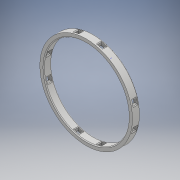
# Autodesk Inventor part: Attache centre
Saved by Autodesk Inventor 2017 (Build 210142000, 142)
## iProperties
Part Number: Attache centre
Material: Générique
Document SubType Name: Modeling
Designer: Thomas
Density: 1 g/cm^3
Appearance: Par défaut
Author: Thomas
Autodesk Inventor part; units mm, degrees
sketch "Esquisse1" plane through (0, 0, 0) normal (0, 1, 0) x (-1, 0, 0)
  line L0 (-42.5, 28) -> (42.5, 28) construction
  line L1 (42.5, 28) -> (42.5, -28) construction
  line L2 (42.5, -28) -> (-42.5, -28) construction
  line L3 (-42.5, -28) -> (-42.5, 28) construction
  line L4 (-42.5, 28) -> (42.5, -28) construction
  line L5 (42.5, 28) -> (-42.5, -28) construction
  circle A0 centre (0, 0) radius 60
  circle A1 centre (0, 0) radius 55
  line L6 (0, 0) -> (94, 94) construction
  line L7 (0, 0) -> (132.9361, 0) construction
  line L8 (0, 0) -> (-94, 94) construction
  line L9 (0, 0) -> (-94, -94) construction
  line L10 (0, 0) -> (94, -94) construction
  arc A2 (42.4264, 42.4264) -> (110, 0) centre (152.2245, 142.2782) ccw construction
  arc A3 (110, 0) -> (42.4264, -42.4264) centre (152.2245, -142.2782) ccw construction
  arc A4 (-42.4264, 42.4264) -> (0, 110) centre (-142.2782, 152.2245) ccw construction
  arc A5 (0, 110) -> (42.4264, 42.4264) centre (142.2782, 152.2245) ccw construction
  arc A6 (-42.4264, -42.4264) -> (-110, 0) centre (-152.2245, -142.2782) ccw construction
  arc A7 (-110, 0) -> (-42.4264, 42.4264) centre (-152.2245, 142.2782) ccw construction
  arc A8 (42.4264, -42.4264) -> (0, -110) centre (142.2782, -152.2245) ccw construction
  arc A9 (0, -110) -> (-42.4264, -42.4264) centre (-142.2782, -152.2245) ccw construction
  arc A10 (-57.9555, 15.5291) -> (-55, 95.2628) centre (-199.3288, 60.6911) ccw construction
  arc A11 (-55, 95.2628) -> (15.5291, 57.9555) centre (47.1043, 202.9694) ccw construction
  arc A12 (15.5291, -57.9555) -> (-55, -95.2628) centre (47.1043, -202.9694) ccw construction
  arc A13 (-55, -95.2628) -> (-57.9555, -15.5291) centre (-199.3288, -60.6911) ccw construction
  line L11 (0, 110) -> (0, 57.9555) construction
  line L12 (-55, -95.2628) -> (0, 0) construction
  line L13 (-55, 95.2628) -> (0, 0) construction
  line L14 (95.3744, -14.2176) -> (35.3744, 89.7054) construction
  line L15 (35.3744, 89.7054) -> (-95.3744, 14.2176) construction
  line L16 (-95.3744, 14.2176) -> (-35.3744, -89.7054) construction
  line L17 (-35.3744, -89.7054) -> (95.3744, -14.2176) construction
  line L18 (95.3744, -14.2176) -> (-95.3744, 14.2176) construction
  line L19 (35.3744, 89.7054) -> (-35.3744, -89.7054) construction
  dimension "d2" = 120
  dimension "d0" = 85
  dimension "d1" = 56
  dimension "d3" = 110
  dimension "d4" = 45
  dimension "d7" = 360
  dimension "d11" = 360
  dimension "d15" = 360
  constraints: 40 end point, 24 point on circle, 13 centre point, 4 midpoint, 4 parallel, 2 coincident, 2 horizontal, 2 perpendicular, 2 point on line, 2 symmetric about line, 1 equal length, 1 vertical, 68 other
  measures "d0" distance of L1.end L2.end
  measures "d1" distance of L0.end L1.end
  measures "d3" diameter of A1
  measures "d4" angle of L7 L6
extrude "Extrusion1" add sketch "Esquisse1" along normal blind 10
ref_plane "Plan de construction1" through (81, 0, 0) normal (1, 0, 0) x (0, 1, 0)
sketch "Esquisse2" plane through (81, 0, 0) normal (1, 0, 0) x (0, 1, 0)
  line L0 (8, 18.0155) -> (2, 18.0155)
  line L1 (2, 18.0155) -> (2, 12.0155)
  line L2 (2, 12.0155) -> (8, 12.0155)
  line L3 (8, 12.0155) -> (8, 18.0155)
  line L4 (8, 18.0155) -> (2, 12.0155) construction
  line L5 (2, 18.0155) -> (8, 12.0155) construction
  line L6 (10.0489, 0.0155) -> (-6.9511, 0.0155) construction
  line L7 (8, -17.9845) -> (2, -17.9845)
  line L8 (2, -17.9845) -> (2, -11.9845)
  line L9 (2, -11.9845) -> (8, -11.9845)
  line L10 (8, -11.9845) -> (8, -17.9845)
  point P0 (0, 0)
  point P1 (5, 15.0155)
  dimension "d22" = 15
  dimension "d26" = 6
  dimension "d27" = 6
  constraints: 22 end point, 4 symmetric about line, 2 horizontal, 2 midpoint, 2 parallel, 1 perpendicular
  measures "d22" distance from line of point (5, 15.015) L6
  measures "d26" distance of L1.end L2.end
  measures "d27" distance of L0.end L1.end
extrude "Extrusion2" cut sketch "Esquisse2" against normal blind 150
ref_plane "Plan de construction2" through (0, 0, 80) normal (0, 0, 1) x (1, 0, 0)
sketch "Esquisse3" plane through (0, 0, 80) normal (0, 0, 1) x (1, 0, 0)
  line L0 (-0.0028, -2.9025) -> (-0.0028, 13.0975) construction
  line L1 (-18.0028, 2) -> (-12.0028, 2)
  line L2 (-12.0028, 2) -> (-12.0028, 8)
  line L3 (-12.0028, 8) -> (-18.0028, 8)
  line L4 (-18.0028, 8) -> (-18.0028, 2)
  line L5 (17.9972, 2) -> (11.9972, 2)
  line L6 (11.9972, 2) -> (11.9972, 8)
  line L7 (11.9972, 8) -> (17.9972, 8)
  line L8 (17.9972, 8) -> (17.9972, 2)
  point P0 (0, 0)
  point P1 (-15.0028, 5)
  point P2 (14.9972, 5)
  dimension "d28" = 6
  dimension "d29" = 6
  dimension "d31" = 15
  dimension "d32" = 3
  dimension "d33" = 3
  constraints: 18 end point, 5 symmetric about line, 2 parallel, 1 horizontal, 1 perpendicular, 1 vertical
  measures "d28" distance of L2.end L3.end
  measures "d29" distance of L3.end L1.start
  measures "d31" distance from line of L0 point (-15.003, 5)
  measures "d32" distance from line of L2 point (-15.003, 5)
  measures "d33" distance from line of L3 point (-15.003, 5)
extrude "Extrusion3" cut sketch "Esquisse3" against normal blind 150
ref_plane "Plan de construction3" through (-35.3744, 0, 89.7054) normal (0.5, 0, 0.866) x (0, 1, 0)
sketch "Esquisse4" plane through (-35.3744, 0, 89.7054) normal (0.5, 0, 0.866) x (0, 1, 0)
  line L0 (0, -75.4878) -> (4, -75.4878) construction
  constraints: 2 end point, 1 horizontal
fillet "Congé1" radius 1 3 edges at (60, 10, 0) (55, 10, 0) (55, 0, 0)
fillet "Congé2" radius 1 32 edges at (-53.6715, 5, 12.0155) (53.6715, 5, 12.0155) (-58.7846, 5, 12.0155) (58.7846, 5, 12.0155) (-57.2315, 5, 18.0155) (57.2315, 5, 18.0155) (-51.9658, 5, 18.0155) (51.9658, 5, 18.0155) (53.6784, 5, -11.9845) (-53.6784, 5, -11.9845) (51.9765, 5, -17.9845) (-51.9765, 5, -17.9845) (57.2412, 5, -17.9845) (-57.2412, 5, -17.9845) (58.7909, 5, -11.9845) (-58.7909, 5, -11.9845) (11.9972, 5, 58.7883) (11.9972, 5, -58.7883) (17.9972, 5, 57.2372) (17.9972, 5, -57.2372) (-18.0028, 5, 51.9702) (-18.0028, 5, -51.9702) (-12.0028, 5, 53.6743) (-12.0028, 5, -53.6743) (11.9972, 5, 53.6756) (11.9972, 5, -53.6756) (17.9972, 5, 51.9721) (17.9972, 5, -51.9721) (-18.0028, 5, 57.2355) (-18.0028, 5, -57.2355) (-12.0028, 5, 58.7872) (-12.0028, 5, -58.7872)
